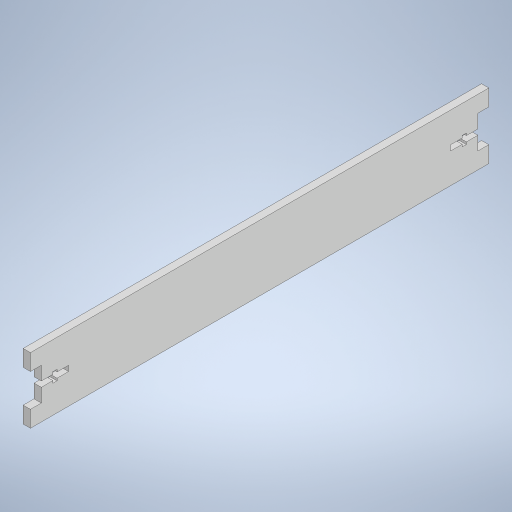
# Autodesk Inventor part: ребро
Saved by Autodesk Inventor 2023.1 (Build 271208000, 208)
## iProperties
Created: 2024-12-25
Part Number: ребро
Material: Типовые
Document SubType Name: Modeling
Designer: DELL
Density: 1 g/cm^3
Appearance: По умолчанию
Author: DELL
Autodesk Inventor part; units mm, degrees
ref_plane "YZ Plane" through (0, 0, 0) normal (1, 0, 0) x (0, 1, 0)
ref_plane "XZ Plane" through (0, 0, 0) normal (0, 1, 0) x (-1, 0, 0)
ref_plane "XY Plane" through (0, 0, 0) normal (0, 0, 1) x (1, 0, 0)
sketch "Эскиз1" plane through (0, 0, 0) normal (0, 0, 1) x (1, 0, 0)
  line L0 (-2, 18) -> (2, 18)
  line L1 (2, -18) -> (-2, -18)
  line L2 (-2, 18) -> (2, -18) construction
  line L3 (2, 18) -> (-2, -18) construction
  line L4 (-2, 9) -> (2, 9)
  line L5 (2, -9) -> (-2, -9)
  line L6 (-2, 9) -> (2, -9) construction
  line L7 (2, 9) -> (-2, -9) construction
  line L8 (-2, -18) -> (-2, -9)
  line L9 (-2, 9) -> (-2, 18)
  line L10 (2, 18) -> (2, 9)
  line L11 (2, -9) -> (2, -18)
  point P0 (0, 0)
  dimension "d4" = 36
  dimension "d5" = 4
  constraints: 24 end point, 6 parallel, 4 midpoint, 2 horizontal, 2 perpendicular
  measures "d4" distance of L1.start L0.end
  measures "d5" distance of L4.start L4.end
extrude "Выдавливание1" add sketch "Эскиз1" along normal blind 6
sketch "Эскиз2" plane through (0, 0, 6) normal (0, 0, 1) x (1, 0, 0)
  line L0 (-2, -18) -> (2, -18) projected
  line L1 (2, 18) -> (-2, 18) projected
  line L2 (-2, -18) -> (2, -18)
  line L3 (2, -18) -> (2, 18)
  line L4 (2, 18) -> (-2, 18)
  line L5 (-2, 18) -> (-2, -18)
  point P0 (0, 0)
  constraints: 8 end point, 2 parallel, 1 horizontal, 1 perpendicular
extrude "Выдавливание2" add sketch "Эскиз2" along normal blind 240
sketch "Эскиз4" plane through (0, 0, 246) normal (0, 0, 1) x (1, 0, 0)
  line L0 (2, 18) -> (-2, 18) projected
  line L1 (-2, -18) -> (2, -18) projected
  line L2 (-2, 18) -> (2, 18)
  line L3 (2, -18) -> (-2, -18)
  line L4 (-2, 9) -> (-2, -9) projected
  line L5 (2, 9) -> (-2, 9)
  line L6 (-2, -9) -> (2, -9)
  line L7 (2, 9) -> (-2, -9) construction
  line L8 (-2, 9) -> (2, -9) construction
  line L9 (2, 18) -> (2, 9)
  line L10 (2, -9) -> (2, -18)
  line L11 (-2, -18) -> (-2, -9)
  line L12 (-2, 9) -> (-2, 18)
  point P0 (0, 0)
  constraints: 20 end point, 6 parallel, 2 horizontal, 2 midpoint, 2 perpendicular
extrude "Выдавливание3" add sketch "Эскиз4" along normal blind 6
sketch "Эскиз5" plane through (-2, -18, 0) normal (-1, 0, 0) x (0, 0, 1)
  line L0 (6, 27) -> (6, 9) projected
  line L1 (231, 19.5) -> (231, 16.5)
  line L2 (246, 19.5) -> (231, 16.5) construction
  line L3 (231, 19.5) -> (246, 16.5) construction
  line L4 (239.65, 20.75) -> (237.35, 20.75)
  line L5 (237.35, 15.25) -> (239.65, 15.25)
  line L6 (239.65, 20.75) -> (237.35, 15.25) construction
  line L7 (237.35, 20.75) -> (239.65, 15.25) construction
  line L8 (246, 19.5) -> (239.65, 19.5)
  line L9 (237.35, 19.5) -> (231, 19.5)
  line L10 (239.65, 15.25) -> (239.65, 16.5)
  line L11 (239.65, 19.5) -> (239.65, 20.75)
  line L12 (231, 16.5) -> (237.35, 16.5)
  line L13 (239.65, 16.5) -> (246, 16.5)
  line L14 (246, 27) -> (246, 19.5)
  line L15 (246, 16.5) -> (246, 9)
  line L16 (0, 0) -> (252, 0) projected
  line L17 (126, -127.9343) -> (126, 327.3325) construction
  line L18 (237.35, 16.5) -> (237.35, 15.25)
  line L19 (237.35, 20.75) -> (237.35, 19.5)
  line L20 (21, 19.5) -> (21, 16.5)
  line L21 (6, 19.5) -> (21, 16.5) construction
  line L22 (21, 19.5) -> (6, 16.5) construction
  line L23 (12.35, 20.75) -> (14.65, 20.75)
  line L24 (14.65, 15.25) -> (12.35, 15.25)
  line L25 (12.35, 20.75) -> (14.65, 15.25) construction
  line L26 (14.65, 20.75) -> (12.35, 15.25) construction
  line L27 (6, 19.5) -> (12.35, 19.5)
  line L28 (14.65, 19.5) -> (21, 19.5)
  line L29 (12.35, 15.25) -> (12.35, 16.5)
  line L30 (12.35, 19.5) -> (12.35, 20.75)
  line L31 (21, 16.5) -> (14.65, 16.5)
  line L32 (12.35, 16.5) -> (6, 16.5)
  line L33 (6, 27) -> (6, 19.5)
  line L34 (6, 16.5) -> (6, 9)
  line L35 (14.65, 16.5) -> (14.65, 15.25)
  line L36 (14.65, 20.75) -> (14.65, 19.5)
  line L37 (246, 19.5) -> (246, 16.5)
  line L38 (246, 27) -> (246, 9) projected
  point P0 (0, 18)
  point P1 (238.5, 18)
  point P2 (246, 18)
  point P3 (126, 0)
  point P4 (13.5, 18)
  point P5 (6, 18)
  dimension "d16" = 5.5
  dimension "d17" = 2.3
  constraints: 72 end point, 14 symmetric about line, 9 parallel, 5 midpoint, 4 perpendicular, 3 horizontal, 1 collinear, 1 point on line, 1 vertical
  measures "d16" distance of L4.end L5.start
  measures "d17" distance of L4.start L4.end
extrude "Выдавливание4" cut sketch "Эскиз5" against normal blind 6
